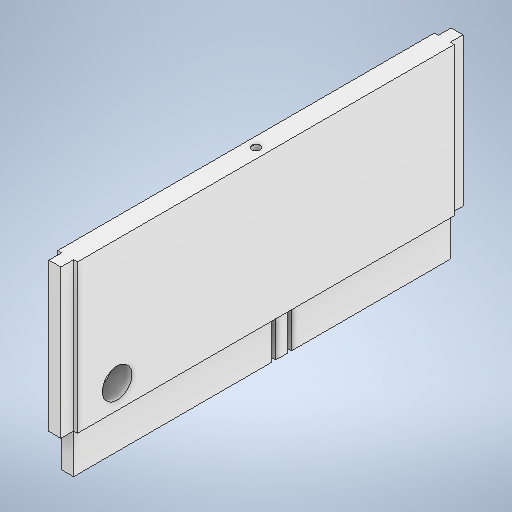
# Autodesk Inventor part: sciana_dluga
Saved by Autodesk Inventor 2025.2 (Build 292293000, 293)
## iProperties
Created: 2026-07-07
Part Number: sciana_dluga
Material: ABS Plastic
Document SubType Name: Modeling
Designer: ksawe
Density: 1.06 g/cm^3
Appearance: Smooth - White
Author: ksawe
Autodesk Inventor part; units mm, degrees
ref_plane "YZ Plane" through (0, 0, 0) normal (1, 0, 0) x (0, 1, 0)
ref_plane "XZ Plane" through (0, 0, 0) normal (0, 1, 0) x (-1, 0, 0)
ref_plane "XY Plane" through (0, 0, 0) normal (0, 0, 1) x (1, 0, 0)
sketch "Sketch1" plane through (0, 0, 0) normal (0, 1, 0) x (-1, 0, 0)
  line L0 (5, 95.202) -> (-5, 95.202)
  line L1 (-5, 95.202) -> (-5, -95.202)
  line L2 (-5, -95.202) -> (5, -95.202)
  line L3 (5, -95.202) -> (5, 95.202)
  line L4 (5, 95.202) -> (-5, -95.202) construction
  line L5 (-5, 95.202) -> (5, -95.202) construction
  line L6 (3, 101.655) -> (-3, 101.655)
  line L7 (-3, 101.655) -> (-3, -101.655)
  line L8 (-3, -101.655) -> (3, -101.655)
  line L9 (3, -101.655) -> (3, 101.655)
  line L10 (3, 101.655) -> (-3, -101.655) construction
  line L11 (-3, 101.655) -> (3, -101.655) construction
  line L12 (-3, -13) -> (3, -13)
  line L13 (3, -13) -> (3, -7)
  line L14 (3, -7) -> (-3, -7)
  line L15 (-3, -7) -> (-3, -13)
  line L16 (-3, -15) -> (3, -15)
  line L17 (3, -5) -> (-3, -5)
  point P0 (0, 0)
  point P1 (0, -7)
  point P2 (-3, -95.202)
  point P3 (3, -95.202)
  point P4 (3, 95.202)
  point P5 (-3, 95.202)
  point P6 (-3, -7)
  dimension "d0" = 10
  dimension "d1" = 190.404
  dimension "d2" = 203.31
  dimension "d4" = 6
  dimension "d5" = 82.202
  dimension "d6" = 6
  dimension "d7" = 6
  dimension "d8" = 2
  dimension "d9" = 2
  constraints: 36 end point, 6 parallel, 5 midpoint, 5 perpendicular, 4 point on line, 3 horizontal, 1 vertical alignment
  measures "d0" distance of L2.end L1.end
  measures "d1" distance between parallel lines of L2 L0
  measures "d2" distance between parallel lines of L8 L6
  measures "d4" distance between parallel lines of L9 L7
  measures "d5" distance between parallel lines of L2 L12
  measures "d6" distance of L12.end L13.end
  measures "d7" distance of L13.end L14.end
  measures "d8" distance between parallel lines of L17 L14
  measures "d9" distance between parallel lines of L12 L16
extrude "Extrusion1" add sketch "Sketch1" along normal blind 75
extrude "Extrusion2" add sketch "Sketch1" against normal blind 20 contours L9 L17 L7 L0 | L2 L7 L16 L9 | L9 L12 L7 L14
sketch "Sketch2" plane through (5, 0, 95.202) normal (1, 0, 0) x (0, 0, -1)
  circle A0 centre (20, 12) radius 7.5
  line L0 (0, 0) -> (0, 75) projected
  line L1 (0, 0) -> (190.404, 0) projected
  point P0 (95.202, 0)
  dimension "d14" = 15
  dimension "d15" = 20
  dimension "d16" = 12
  constraints: 1 centre point
  measures "d14" diameter of A0
  measures "d15" distance from line of L0 A0.centre
  measures "d16" distance from line of L1 A0.centre
extrude "Extrusion3" cut sketch "Sketch2" against normal blind 75
sketch "Sketch3" plane through (0, 75, 0) normal (0, 1, 0) x (1, 0, 0)
  line L0 (-3, -101.655) -> (3, -101.655) projected
  line L1 (-5, 95.202) -> (-5, -95.202) projected
  point P0 (0, 0)
  point P1 (0, 0)
  dimension "d26" = 101.655
  dimension "d27" = 5
  measures "d26" distance from line of L0 point (0, 0)
  measures "d27" distance from line of L1 point (0, 0)
hole "Hole1" at (0, 75, 0) direction (0, -1, 0) diameter 4 depth 7 countersink diameter 4.2 countersink angle 90
sketch "Sketch4" plane through (0, -20, 0) normal (0, -1, 0) x (1, 0, 0)
  line L0 (3, -13) -> (3, -7) projected
  point P0 (0, 0)
  point P1 (0, -9.8779)
  dimension "d28" = 3
  measures "d28" distance from line of L0 point (0, -9.878)
hole "Hole2" at (0, -20, -9.8779) direction (0, 1, 0) diameter 4 depth 7 countersink diameter 4.2 countersink angle 90
body "Solid1"
